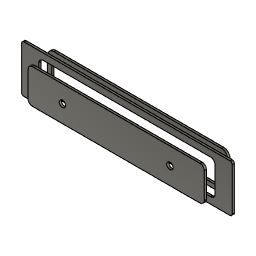
MEDIAbay (Autodesk Fusion 360 design; units mm, degrees)
Autodesk Fusion 360 part; units mm, degrees
sketch "Sketch1" plane through (0, 0, 0) normal (0, 1, 0) x (1, 0, 0)
  line L0 (480, -110) -> (-480, -110)
  line L1 (-490, -100) -> (-490, 100)
  line L2 (-480, 110) -> (480, 110)
  line L3 (490, 100) -> (490, -100)
  line L4 (490, -110) -> (-490, 110) construction
  line L5 (-490, -110) -> (490, 110) construction
  arc A0 (480, -110) -> (490, -100) centre (480, -100) ccw
  arc A1 (490, 100) -> (480, 110) centre (480, 100) ccw
  arc A2 (-480, 110) -> (-490, 100) centre (-480, 100) ccw
  arc A3 (-490, -100) -> (-480, -110) centre (-480, -100) ccw
  line L6 (390, 80) -> (-390, 80)
  line L7 (-410, 60) -> (-410, -60)
  line L8 (-390, -80) -> (390, -80)
  line L9 (410, -60) -> (410, 60)
  line L10 (410, 80) -> (-410, -80) construction
  line L11 (-410, 80) -> (410, -80) construction
  arc A4 (390, -80) -> (410, -60) centre (390, -60) ccw
  arc A5 (410, 60) -> (390, 80) centre (390, 60) ccw
  arc A6 (-390, 80) -> (-410, 60) centre (-390, 60) ccw
  arc A7 (-410, -60) -> (-390, -80) centre (-390, -60) ccw
  line L12 (-650, 0) -> (650, 0) construction
  line L13 (0, -300) -> (0, 250) construction
  circle A8 centre (250, 0) radius 15
  circle A9 centre (-250, 0) radius 15
  arc A10 (420, 60) -> (390, 90) centre (390, 60) ccw
  line L14 (390, 90) -> (-390, 90)
  arc A11 (-390, 90) -> (-420, 60) centre (-390, 60) ccw
  line L15 (-420, 60) -> (-420, -60)
  arc A12 (-420, -60) -> (-390, -90) centre (-390, -60) ccw
  line L16 (-390, -90) -> (390, -90)
  arc A13 (390, -90) -> (420, -60) centre (390, -60) ccw
  line L17 (420, -60) -> (420, 60)
  arc A14 (400, 60) -> (390, 70) centre (390, 60) ccw
  line L18 (390, 70) -> (-390, 70)
  arc A15 (-390, 70) -> (-400, 60) centre (-390, 60) ccw
  line L19 (-400, 60) -> (-400, -60)
  arc A16 (-400, -60) -> (-390, -70) centre (-390, -60) ccw
  line L20 (-390, -70) -> (390, -70)
  arc A17 (390, -70) -> (400, -60) centre (390, -60) ccw
  line L21 (400, -60) -> (400, 60)
  dimension "d1" = 980
  dimension "d2" = 220
  dimension "d3" = 10
  dimension "d4" = 10
  dimension "d5" = 10
  dimension "d6" = 10
  dimension "d7" = 820
  dimension "d8" = 160
  dimension "d9" = 20
  dimension "d10" = 20
  dimension "d11" = 20
  dimension "d12" = 20
  dimension "d15" = 1300
  dimension "d16" = 550
  dimension "d17" = 30
  dimension "d18" = 80
  dimension "d19" = 250
  dimension "d23" = 10
  dimension "d24" = -10
  constraint horizontal L0
  constraint perpendicular L0 L1
  constraint parallel L0 L2
  constraint parallel L1 L3
  constraint coincident L4 origin
  constraint coincident L5 origin
  constraint coincident L4.start L0
  constraint coincident L4.start L3
  constraint tangent L0 A0
  constraint tangent L3 A0
  constraint coincident L5.end L3
  constraint coincident L5.end L2
  constraint tangent L3 A1
  constraint tangent L2 A1
  constraint coincident L4.end L2
  constraint coincident L4.end L1
  constraint tangent L2 A2
  constraint tangent L1 A2
  constraint coincident L5.start L1
  constraint coincident L5.start L0
  constraint tangent L1 A3
  constraint tangent L0 A3
  constraint horizontal L6
  constraint perpendicular L6 L7
  constraint parallel L6 L8
  constraint parallel L7 L9
  constraint coincident L10 origin
  constraint coincident L11 origin
  constraint coincident L11.end L8
  constraint coincident L11.end L9
  constraint tangent L8 A4
  constraint tangent L9 A4
  constraint coincident L10.start L9
  constraint coincident L10.start L6
  constraint tangent L9 A5
  constraint tangent L6 A5
  constraint coincident L11.start L6
  constraint coincident L11.start L7
  constraint tangent L6 A6
  constraint tangent L7 A6
  constraint coincident L10.end L7
  constraint coincident L10.end L8
  constraint tangent L7 A7
  constraint tangent L8 A7
  constraint horizontal L12
  constraint perpendicular L2 L13
  constraint coincident L12 A8.centre
  constraint symmetric L13 A8 A9
  measures "d1" distance of L4.end L5.end
  measures "d2" distance of L5.start L4.end
  measures "d3" radius of A0
  measures "d4" radius of A1
  measures "d5" radius of A2
  measures "d6" radius of A3
  measures "d7" distance of L10.end L11.end
  measures "d8" distance of L11.start L10.end
  measures "d9" radius of A4
  measures "d10" radius of A5
  measures "d11" radius of A6
  measures "d12" radius of A7
  measures "d15" distance of L12.start L12.end
  measures "d16" distance of L13.start L13.end
  measures "d17" diameter of A8
  measures "d18" distance of L6 A8.centre
  measures "d19" distance of origin A8.centre
extrude "Extrude1" add sketch "Sketch1" along normal blind 10 contours L0 L1 L2 L3 A0 A1 A2 A3 | A10 L14 A11 L15 A12 L16 A13 L17 makes body 1 in component "Frame"
extrude "Extrude1'" add sketch "Sketch1" along normal blind 10 from surface at -50 separate body contours L6 L7 L8 L9 A4 A5 A6 A7 | A14 L18 A15 L19 A16 L20 A17 L21 makes body 2 in component "Door"
extrude "Extrude1''" add sketch "Sketch1" along normal blind 10 from surface at 50 separate body contours L6 L7 L8 L9 A4 A5 A6 A7 | A10 L14 A11 L15 A12 L16 A13 L17 makes body 3 in component "Rim"
component "Frame" placed x (1, 0, 0) y (0, 1, 0) z (0, 0, 1) at (0, 0, 0)
component "Door" placed x (1, 0, 0) y (0, 1, 0) z (0, 0, 1) at (0, 0, 0)
component "Rim" placed x (1, 0, 0) y (0, 1, 0) z (0, 0, 1) at (0, 0, 0)
